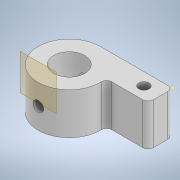
# Autodesk Inventor part: Assignment 2.6 - Shaft Guide
Saved by Autodesk Inventor 2022 (Build 260153000, 153)
## iProperties
Created: 2021-05-23
Part Number: Assignment 2.6 - Shaft Guide
Material: Generic
Document SubType Name: Modeling
Designer: Aaron
Density: 1 g/cm^3
Appearance: Default
Author: Aaron
Autodesk Inventor part; units mm, degrees
ref_plane "YZ Plane" through (0, 0, 0) normal (1, 0, 0) x (0, 1, 0)
ref_plane "XZ Plane" through (0, 0, 0) normal (0, 1, 0) x (-1, 0, 0)
ref_plane "XY Plane" through (0, 0, 0) normal (0, 0, 1) x (1, 0, 0)
sketch "Sketch1" plane through (0, 0, 0) normal (0, 0, 1) x (1, 0, 0)
  point P0 (0, 0)
sketch "Sketch2" plane through (0, 0, 0) normal (0, 1, 0) x (-1, 0, 0)
  line L0 (3.175, 0) -> (44.45, 0)
  circle A0 centre (44.45, 19.05) radius 9.525
  arc A1 (44.45, 0) -> (25.4113, 18.3929) centre (44.45, 19.05) ccw
  line L1 (0, 3.175) -> (0, 12.065)
  circle A2 centre (10.16, 7.62) radius 3.175
  line L2 (3.175, 15.24) -> (22.6099, 15.24)
  arc A3 (3.175, 15.24) -> (0, 12.065) centre (3.175, 12.065) ccw
  arc A4 (0, 3.175) -> (3.175, 0) centre (3.175, 3.175) ccw
  arc A5 (22.6099, 15.24) -> (25.4113, 18.3929) centre (22.2363, 18.3929) ccw
  point P0 (0, 0)
  point P1 (0, 15.24)
  dimension "d1" = 44.45
  dimension "d3" = 19.05
  dimension "d4" = 38.1
  dimension "d5" = 15.24
  dimension "d7" = 6.35
  dimension "d8" = 3.175
  dimension "d11" = 3.175
  constraints: 8 point on circle, 6 centre point, 6 end point, 4 point on line, 4 tangent, 2 horizontal, 1 coincident, 1 equal radius, 1 vertical
  measures "d1" distance of L0.end point (0, 0)
  measures "d3" diameter of A0
  measures "d4" diameter of A1
  measures "d5" distance of point (0, 0) point (0, 15.24)
  measures "d7" diameter of A2
  measures "d8" radius of A3
  measures "d11" radius of A5
extrude "Extrusion1" add sketch "Sketch2" against normal blind 25.4
ref_plane "Work Plane5" through (-44.45, 0, 38.1) normal (0, 0, 1) x (1, 0, 0)
sketch "Sketch5" plane through (-44.45, 0, 38.1) normal (0, 0, 1) x (1, 0, 0)
  line L0 (-19.05, 0) -> (-19.05, -25.4) projected
  circle A0 centre (0, -12.7) radius 3.175
  point P0 (44.45, 0)
  point P1 (0, -25.4)
  point P2 (19.0387, -25.4)
  dimension "d21" = 6.35
  constraints: 1 centre point, 1 point on line
  measures "d21" diameter of A0
extrude "Extrusion2" cut sketch "Sketch5" against normal through all
body "Solid1"
